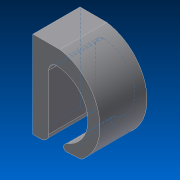
# Autodesk Inventor part: cable hook 5mm-2mm opening
Saved by Autodesk Inventor 2015 (Build 190159000, 159)
## iProperties
Created: 2017-03-25
Part Number: cable hook 5mm-2mm opening
Material: Generic
Document SubType Name: Modeling
Designer: ZigZagJoe
Density: 1 g/cm^3
Appearance: Default
Author: ZigZagJoe
Autodesk Inventor part; units mm, degrees
ref_plane "YZ Plane" through (0, 0, 0) normal (1, 0, 0) x (0, 1, 0)
ref_plane "XZ Plane" through (0, 0, 0) normal (0, 1, 0) x (-1, 0, 0)
ref_plane "XY Plane" through (0, 0, 0) normal (0, 0, 1) x (1, 0, 0)
sketch "Sketch1" plane through (0, 0, 0) normal (0, 1, 0) x (-1, 0, 0)
  line L0 (4.9223, 0.8124) -> (4.9223, -5.2521)
  line L1 (5.9223, -6.2521) -> (6.9223, -6.2521)
  line L2 (6.9223, -6.2521) -> (6.9223, 4.8364)
  line L3 (6.9223, 4.8364) -> (3.5067, 4.8364)
  arc A0 (3.5067, 4.8364) -> (0.6365, -5.8307) centre (4.4005, -1.1238) ccw
  arc A1 (4.0891, 2.8364) -> (2.4729, -5.0213) centre (4, -1.2403) ccw
  arc A2 (2.9716, -5.4611) -> (2.4729, -5.0213) centre (2.0984, -5.9485) ccw
  arc A3 (4.9223, -5.2521) -> (5.9223, -6.2521) centre (5.9223, -5.2521) ccw
  line L4 (4.9223, 0.8124) -> (4.9223, 1.8364)
  line L5 (3.9223, 2.8364) -> (4.0891, 2.8364)
  arc A4 (4.9223, 1.8364) -> (3.9223, 2.8364) centre (3.9223, 1.8364) ccw
  line L6 (0.8547, -5.917) -> (2.5906, -6.0548)
  arc A5 (2.5906, -6.0548) -> (2.9716, -5.4611) centre (2.6223, -5.656) ccw
  arc A6 (0.6365, -5.8307) -> (0.8547, -5.917) centre (0.8864, -5.5183) ccw
  point P0 (0, 0)
  point P1 (4.9223, -6.2521)
  point P2 (2.9653, -6.9772)
  point P3 (2.8675, -5.1576)
  point P4 (3.0877, -6.0942)
  point P5 (0.7347, -5.9075)
  dimension "d1" = 2
  dimension "d5" = 1
  dimension "d7" = 5
  dimension "d8" = 1
  dimension "d9" = 2
  dimension "d10" = 1
  dimension "d13" = 0.4
  dimension "d14" = 2.3
  constraints: 19 point on circle, 14 end point, 9 tangent, 7 centre point, 4 perpendicular, 4 point on line, 2 vertical, 1 equal radius
  measures "d1" distance of point (4.922, -6.252) L1.end
  measures "d5" radius of A2
  measures "d8" radius of A3
  measures "d9" distance between parallel lines of L3 L5
  measures "d10" radius of A4
  measures "d13" radius of A5
  measures "d14" distance from line of L0 A5.centre
extrude "Extrusion1" add sketch "Sketch1" along normal blind 6
body "Solid1"
